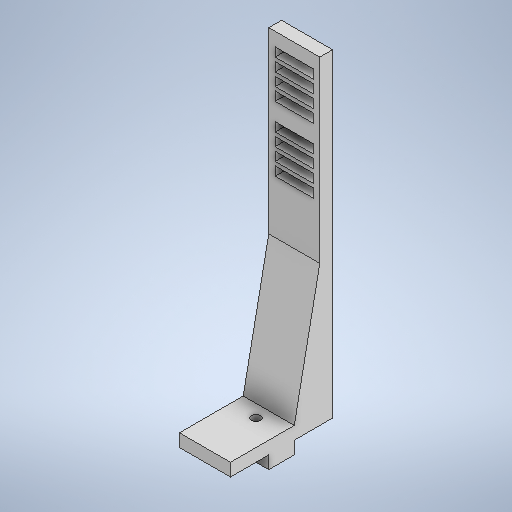
# Autodesk Inventor part: Indu_Holder
Saved by Autodesk Inventor 2025.2 (Build 292293000, 293)
## iProperties
Created: 2025-05-10
Part Number: Indu_Holder
Material: Generic
Document SubType Name: Modeling
Designer: lauri
Density: 1 g/cm^3
Appearance: Default
Author: lauri
Autodesk Inventor part; units mm, degrees
ref_plane "YZ Plane" through (0, 0, 0) normal (1, 0, 0) x (0, 1, 0)
ref_plane "XZ Plane" through (0, 0, 0) normal (0, 1, 0) x (-1, 0, 0)
ref_plane "XY Plane" through (0, 0, 0) normal (0, 0, 1) x (1, 0, 0)
sketch "Sketch1" plane through (0, 0, 0) normal (0, 1, 0) x (-1, 0, 0)
  line L0 (-10, 5) -> (10, 5)
  line L1 (10, 5) -> (10, -5)
  line L2 (10, -5) -> (-10, -5)
  line L3 (-10, -5) -> (-10, 5)
  line L4 (-10, 5) -> (10, -5) construction
  line L5 (10, 5) -> (-10, -5) construction
  point P0 (0, 0)
  dimension "d0" = 20
  dimension "d1" = 10
  constraints: 12 end point, 2 midpoint, 2 parallel, 1 horizontal, 1 perpendicular
  measures "d0" distance of L1.end L2.end
  measures "d1" distance of L0.end L1.end
extrude "Extrusion1" add sketch "Sketch1" along normal blind 5
sketch "Sketch7" plane through (0, 5, 0) normal (0, 1, 0) x (1, 0, 0)
  line L0 (10, -20) -> (-10, -20)
  line L1 (-10, -20) -> (-10, 20)
  line L2 (-10, 20) -> (10, 20)
  line L3 (10, 20) -> (10, -20)
  line L4 (10, -20) -> (-10, 20) construction
  line L5 (-10, -20) -> (10, 20) construction
  point P0 (0, 0)
  dimension "d26" = 40
  constraints: 12 end point, 2 midpoint, 2 parallel, 1 horizontal, 1 perpendicular
  measures "d26" distance of L0.end L1.end
extrude "Extrusion4" add sketch "Sketch7" along normal blind 5
sketch "Sketch8" plane through (0, 10, 0) normal (0, 1, 0) x (1, 0, 0)
  line L0 (10, 20) -> (-10, 20) projected
  line L1 (10, 5) -> (10, 20) projected
  line L2 (-10, 20) -> (10, 20)
  line L3 (10, 20) -> (10, 15)
  line L4 (10, 15) -> (-10, 15)
  line L5 (-10, 15) -> (-10, 20)
  point P0 (0, 0)
  dimension "d29" = 5
  constraints: 8 end point, 2 parallel, 1 horizontal, 1 perpendicular, 1 point on line
  measures "d29" distance of L2.end L3.end
extrude "Extrusion5" add sketch "Sketch8" along normal blind 120
sketch "Sketch9" plane through (0, 10, 0) normal (0, 1, 0) x (1, 0, 0)
  line L0 (10, 15) -> (-10, 15) projected
  line L1 (10, -20) -> (10, 15) projected
  line L2 (-10, 15) -> (10, 15)
  line L3 (10, 15) -> (10, 5)
  line L4 (10, 5) -> (-10, 5)
  line L5 (-10, 5) -> (-10, 15)
  point P0 (0, 0)
  dimension "d32" = 10
  constraints: 8 end point, 2 parallel, 1 horizontal, 1 perpendicular, 1 point on line
  measures "d32" distance of L2.end L3.end
extrude "Extrusion6" add sketch "Sketch9" along normal blind 50
chamfer "Chamfer1" distance 10 distance2 50 1 edges at (0, 60, -5) measured on face at (-3.3333, 60, -11.6667)
sketch "Sketch10" plane through (0, 10, 0) normal (0, 1, 0) x (1, 0, 0)
  point P0 (0, 0)
  point P1 (0, 0)
  constraints: 1 coincident
hole "Hole3" at (0, 10, 0) direction (0, -1, 0) diameter 3.5 depth 10
sketch "Sketch11" plane through (-10, 130, -15) normal (0, 0, 1) x (1, 0, 0)
  line L0 (2.5, -8.75) -> (17.5, -8.75)
  line L1 (17.5, -8.75) -> (17.5, -5.25)
  line L2 (17.5, -5.25) -> (2.5, -5.25)
  line L3 (2.5, -5.25) -> (2.5, -8.75)
  line L4 (2.5, -8.75) -> (17.5, -5.25) construction
  line L5 (17.5, -8.75) -> (2.5, -5.25) construction
  line L6 (2.5, -10.25) -> (17.5, -10.25)
  line L7 (17.5, -10.25) -> (17.5, -13.75)
  line L8 (17.5, -13.75) -> (2.5, -13.75)
  line L9 (2.5, -13.75) -> (2.5, -10.25)
  line L10 (2.5, -10.25) -> (17.5, -13.75) construction
  line L11 (17.5, -10.25) -> (2.5, -13.75) construction
  line L12 (2.5, -15.25) -> (17.5, -15.25)
  line L13 (17.5, -15.25) -> (17.5, -18.75)
  line L14 (17.5, -18.75) -> (2.5, -18.75)
  line L15 (2.5, -18.75) -> (2.5, -15.25)
  line L16 (2.5, -15.25) -> (17.5, -18.75) construction
  line L17 (17.5, -15.25) -> (2.5, -18.75) construction
  line L18 (2.5, -23.75) -> (17.5, -23.75)
  line L19 (17.5, -23.75) -> (17.5, -20.25)
  line L20 (17.5, -20.25) -> (2.5, -20.25)
  line L21 (2.5, -20.25) -> (2.5, -23.75)
  line L22 (2.5, -23.75) -> (17.5, -20.25) construction
  line L23 (17.5, -23.75) -> (2.5, -20.25) construction
  line L24 (2.5, -34.15) -> (17.5, -34.15)
  line L25 (17.5, -34.15) -> (17.5, -30.65)
  line L26 (17.5, -30.65) -> (2.5, -30.65)
  line L27 (2.5, -30.65) -> (2.5, -34.15)
  line L28 (2.5, -34.15) -> (17.5, -30.65) construction
  line L29 (17.5, -34.15) -> (2.5, -30.65) construction
  line L30 (2.5, -39.15) -> (17.5, -39.15)
  line L31 (17.5, -39.15) -> (17.5, -35.65)
  line L32 (17.5, -35.65) -> (2.5, -35.65)
  line L33 (2.5, -35.65) -> (2.5, -39.15)
  line L34 (2.5, -39.15) -> (17.5, -35.65) construction
  line L35 (17.5, -39.15) -> (2.5, -35.65) construction
  line L36 (2.5, -44.15) -> (17.5, -44.15)
  line L37 (17.5, -44.15) -> (17.5, -40.65)
  line L38 (17.5, -40.65) -> (2.5, -40.65)
  line L39 (2.5, -40.65) -> (2.5, -44.15)
  line L40 (2.5, -44.15) -> (17.5, -40.65) construction
  line L41 (17.5, -44.15) -> (2.5, -40.65) construction
  line L42 (2.5, -49.15) -> (17.5, -49.15)
  line L43 (17.5, -49.15) -> (17.5, -45.65)
  line L44 (17.5, -45.65) -> (2.5, -45.65)
  line L45 (2.5, -45.65) -> (2.5, -49.15)
  line L46 (2.5, -49.15) -> (17.5, -45.65) construction
  line L47 (17.5, -49.15) -> (2.5, -45.65) construction
  point P0 (10, -130)
  point P1 (10, -7)
  point P2 (10, -32.4)
  point P3 (10, -12)
  point P4 (10, -37.4)
  point P5 (10, -17)
  point P6 (10, -42.4)
  point P7 (10, -22)
  point P8 (10, -47.4)
  dimension "d52" = 15
  dimension "d53" = 3.5
  dimension "d54" = 3.5
  dimension "d55" = 3.5
  dimension "d56" = 3.5
  dimension "d57" = 3.5
  dimension "d58" = 3.5
  dimension "d59" = 3.5
  dimension "d60" = 3.5
  constraints: 96 end point, 16 midpoint, 16 parallel, 8 horizontal, 8 perpendicular, 7 point on line
  measures "d52" distance of L2.end L1.end
  measures "d53" distance of L1.end L0.end
  measures "d54" distance of L6.end L7.end
  measures "d55" distance of L12.end L13.end
  measures "d56" distance of L19.end L18.end
  measures "d57" distance of L25.end L24.end
  measures "d58" distance of L31.end L30.end
  measures "d59" distance of L37.end L36.end
  measures "d60" distance of L43.end L42.end
extrude "Extrusion7" cut sketch "Sketch11" against normal through all
body "Solid1"
